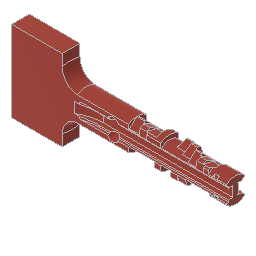
disklock family (Autodesk Fusion 360 design; units mm, degrees)
Autodesk Fusion 360 part; units mm, degrees
sketch "full profile" plane through (0, 0, 0) normal (0, 1, 0) x (1, 0, 0)
  circle A0 centre (0, 0) radius 2.98 construction
  line L0 (0, 0) -> (1.75, 0) construction
  line L1 (0, 0) -> (-1.75, 0) construction
  line L2 (1.75, 0) -> (1.75, -2.412)
  line L3 (1.75, 0) -> (1.75, 2.412)
  line L4 (-1.75, 0) -> (-1.75, 2.412)
  line L5 (-1.75, 0) -> (-1.75, -2.412)
  arc A1 (-1.75, -2.412) -> (1.75, -2.412) centre (0, 0) ccw
  arc A2 (1.75, 2.412) -> (-1.75, 2.412) centre (0, 0) ccw
  dimension "d1" = 5.96
  dimension "d2" = 1.75
  dimension "d3" = 1.75
  constraint coincident A0.centre L0.start
  constraint horizontal L0
  constraint parallel L0 L1
  constraint coincident A0 L2.end
  constraint perpendicular L0 L2
  constraint coincident A0 L3.end
  constraint perpendicular L0 L3
  constraint coincident A0 L4.end
  constraint perpendicular L1 L4
  constraint coincident A0 L5.end
  constraint perpendicular L1 L5
  measures "d1" diameter of A0
  measures "d2" distance of A0.centre L0.end
  measures "d3" distance of A0.centre L1.end
extrude "blade extrude" add sketch "full profile" along normal blind 32.5 makes body 1
sketch "bearing align" plane through (-1.75, 0, 0) normal (-1, 0, 0) x (0, -1, 0)
  line L0 (0, -2.412) -> (0, 2.412)
  line L1 (0, 2.412) -> (-32.5, 2.412)
  line L2 (-32.5, 2.412) -> (-32.5, -2.412)
  line L3 (-32.5, -2.412) -> (0, -2.412)
  line L4 (0, 0) -> (-22.5, 0) construction
  line L5 (-22.5, 0) -> (-22.5, 1) construction
  dimension "d6" = 22.5
  dimension "d7" = 1
  constraint coincident L4.start origin
  constraint perpendicular L0 L4
  constraint perpendicular L4 L5
  measures "d6" distance of L4.start L4.end
  measures "d7" distance of L4.end L5.end
sketch "bearings" plane through (0, 0, 0) normal (0, -1, 0) x (1, 0, 0)
  line L0 (1.75, -2.412) -> (1.75, 2.412)
  arc A0 (1.75, 2.412) -> (-1.75, 2.412) centre (0, 0) ccw
  line L1 (-1.75, 2.412) -> (-1.75, -2.412)
  arc A1 (-1.75, -2.412) -> (1.75, -2.412) centre (0, 0) ccw
  line L2 (1.75, 0) -> (-3.19, 0) construction
  line L3 (-3.19, 0) -> (-3.19, 1) construction
  line L4 (-3.19, 1) -> (-1.9994, 1)
  circle A2 centre (-1.9994, 1) radius 1.1906
  line L5 (-3.19, 0) -> (-3.19, -1) construction
  line L6 (-3.19, -1) -> (-1.9994, -1)
  circle A3 centre (-1.9994, -1) radius 1.1906
  line L7 (-1.9994, 1) -> (-0.8087, 1)
  line L8 (-1.9994, -1) -> (-0.8087, -1)
  dimension "d8" = 4.94
  dimension "d9" = 1
  dimension "d10" = 1.1906
  dimension "d11" = 2.3813
  dimension "d12" = 1
  dimension "d13" = 1.1906
  dimension "d14" = 2.3813
  constraint midpoint L0 L2.start
  constraint perpendicular L0 L2
  constraint perpendicular L2 L3
  constraint perpendicular L3 L4
  constraint coincident L4.end A2.centre
  constraint perpendicular L2 L5
  constraint perpendicular L5 L6
  constraint coincident L6.end A3.centre
  constraint coincident A2 L7.end
  constraint perpendicular L1 L7
  constraint coincident A3 L8.end
  constraint perpendicular L1 L8
  measures "d8" distance of L2.start L2.end
  measures "d9" distance of L2.end L3.end
  measures "d10" distance of L3.end L4.end
  measures "d11" diameter of A2
  measures "d12" distance of L2.end L5.end
  measures "d13" distance of L5.end L6.end
  measures "d14" diameter of A3
revolve "bearing 1 revolve" add sketch "bearings" angle 360 about axis through (-1.9994, 0, 1) along (1, 0, 0) separate body contours L1 A2 L7 | L1 L4 A2 L7 makes body 2
revolve "bearing 2 revolve" add sketch "bearings" angle 360 about axis through (-3.19, 0, -1) along (1, 0, 0) separate body contours L1 L6 A3 L8 | L1 A3 L8 makes body 3
move_body "bearing move" bodies 2 3 to x (1, 0, 0) y (0, 1, 0) z (0, 0, 1) at (0, 22.5, 0)
mirror "bearing mirror" about plane through (0, 0, 0) normal (1, 0, 0) of bodies 2 3 makes body 4 at (2.0624, 23.5297, 0.4055) makes body 5 at (2.0624, 22.6243, 0.1824)
combine "dimple cuts" operation cut target body 1 tool bodies 2 3 4 5
sketch "keyway profile" plane through (0, 0, 0) normal (0, -1, 0) x (1, 0, 0)
  line L0 (1.75, -2.412) -> (1.75, 2.412)
  arc A0 (1.75, 2.412) -> (-1.75, 2.412) centre (0, 0) ccw
  line L1 (-1.75, 2.412) -> (-1.75, -2.412)
  arc A1 (-1.75, -2.412) -> (1.75, -2.412) centre (0, 0) ccw
  line L2 (0, 0) -> (0.5, 0) construction
  line L3 (0.5, 0) -> (0.5, 1.035)
  line L4 (0.5, 1.035) -> (1.75, 1.035)
  line L5 (0.5, 0) -> (0.5, -1.035)
  line L6 (0.5, -1.035) -> (1.75, -1.035)
  line L7 (0, 0) -> (-0.5, 0) construction
  line L8 (-0.5, 0) -> (-0.5, 1.035)
  line L9 (-0.5, 0) -> (-0.5, -1.035)
  line L10 (-0.5, -1.035) -> (-1.75, -1.035)
  line L11 (-0.5, 1.035) -> (-1.75, 1.035)
  dimension "d22" = 0.5
  dimension "d23" = 1.035
  dimension "d24" = 1.035
  dimension "d25" = 0.5
  dimension "d26" = 1.035
  dimension "d27" = 1.035
  constraint coincident A0.centre A1.centre
  constraint perpendicular L1 L2
  constraint perpendicular L2 L3
  constraint coincident L0 L4.end
  constraint perpendicular L0 L4
  constraint perpendicular L2 L5
  constraint coincident L0 L6.end
  constraint perpendicular L0 L6
  constraint parallel L2 L7
  constraint perpendicular L7 L8
  constraint perpendicular L7 L9
  constraint coincident L1 L10.end
  constraint perpendicular L1 L10
  constraint coincident L1 L11.end
  constraint perpendicular L1 L11
  measures "d22" distance of A0.centre L2.end
  measures "d23" distance of L2.end L3.end
  measures "d24" distance of L2.end L5.end
  measures "d25" distance of A0.centre L7.end
  measures "d26" distance of L7.end L8.end
  measures "d27" distance of L7.end L9.end
extrude "keyway profile cut" cut sketch "keyway profile" against normal blind 30 contours L0 L3 L4 L5 L6 | L1 L8 L9 L10 L11 bodies 1
fillet "Fillet2" radius 8.5 2 edges at (-0.5, 30, 0) (0.5, 30, 0) on bodies 1
sketch "novel spinner warding" plane through (0, 0, 0) normal (0, 1, 0) x (1, 0, 0)
  line L0 (0, 0) -> (1.75, 0) construction
  line L1 (1.75, 0) -> (1.75, 0.99) construction
  line L2 (1.75, 0.99) -> (1.3741, 0.99)
  line L3 (1.3741, 0.99) -> (1.3741, 1.3518)
  line L4 (1.75, 0.99) -> (1.75, 1.4886)
  line L5 (1.75, 1.4886) -> (1.3741, 1.3518)
  line L6 (0, 0) -> (-1.75, 0) construction
  line L7 (-1.75, 0) -> (-1.75, -0.99) construction
  line L8 (-1.75, -0.99) -> (-1.3741, -0.99)
  line L9 (-1.3741, -0.99) -> (-1.3741, -1.3518)
  line L10 (-1.75, -0.99) -> (-1.75, -1.4886)
  line L11 (-1.75, -1.4886) -> (-1.3741, -1.3518)
  line L12 (0, 0) -> (0, 1.75) construction
  line L13 (1.3741, -0.99) -> (1.3741, -1.3518)
  line L14 (1.75, -0.99) -> (1.3741, -0.99)
  line L15 (1.75, -0.99) -> (1.75, -1.4886)
  line L16 (1.75, -1.4886) -> (1.3741, -1.3518)
  line L17 (-1.75, 1.4886) -> (-1.3741, 1.3518)
  line L18 (-1.75, 0.99) -> (-1.75, 1.4886)
  line L19 (-1.3741, 0.99) -> (-1.3741, 1.3518)
  line L20 (-1.75, 0.99) -> (-1.3741, 0.99)
  dimension "d30" = 1.75
  dimension "d31" = 0.99
  dimension "d32" = 0.3759
  dimension "d33" = 0.3618
  dimension "d34" = 0.4986
  dimension "d35" = 1.75
  dimension "d36" = 0.99
  dimension "d37" = 0.3759
  dimension "d38" = 0.3618
  dimension "d39" = 0.4986
  dimension "d40" = 1.75
  constraint coincident L0.start L6.start
  constraint horizontal L0
  constraint perpendicular L0 L1
  constraint perpendicular L1 L2
  constraint perpendicular L2 L3
  constraint perpendicular L2 L4
  constraint parallel L0 L6
  constraint perpendicular L6 L7
  constraint perpendicular L7 L8
  constraint perpendicular L8 L9
  constraint perpendicular L8 L10
  constraint perpendicular L6 L12
  constraint symmetric L1.end L12 L18.start
  constraint symmetric L2.end L12 L19.start
  constraint symmetric L3.end L12 L17.end
  constraint symmetric L4.end L12 L17.start
  constraint symmetric L7.end L12 L14.start
  constraint symmetric L8.end L12 L13.start
  constraint symmetric L9.end L12 L13.end
  constraint symmetric L10.end L12 L15.end
  measures "d30" distance of L0.start L0.end
  measures "d31" distance of L0.end L1.end
  measures "d32" distance of L1.end L2.end
  measures "d33" distance of L2.end L3.end
  measures "d34" distance of L1.end L4.end
  measures "d35" distance of L0.start L6.end
  measures "d36" distance of L6.end L7.end
  measures "d37" distance of L7.end L8.end
  measures "d38" distance of L8.end L9.end
  measures "d39" distance of L7.end L10.end
  measures "d40" distance of L0.start L12.end
extrude "spinner warding cut" cut sketch "novel spinner warding" along normal blind 29 bodies 1
fillet "Fillet1" radius 15.9 4 edges at (1.3741, 29, -1.1934) (1.3741, 29, 1.1934) (-1.3741, 29, 1.1934) (-1.3741, 29, -1.1934) on bodies 1
sketch "driver plate cut" plane through (0, 0, 0) normal (0, 1, 0) x (1, 0, 0)
  circle A0 centre (0, 0) radius 3.15 construction
  line L0 (0, 0) -> (1.82, 0) construction
  line L1 (0, 0) -> (1.758, -0.4711) construction
  line L2 (0, 0) -> (1.82, 0) construction
  line L3 (1.758, -0.4711) -> (1.0926, -2.9545)
  line L4 (0, 0) -> (-1.82, 0) construction
  line L5 (0, 0) -> (-1.758, 0.4711) construction
  line L6 (0, 0) -> (1.758, 0.4711) construction
  line L7 (0, 0) -> (1.82, 0) construction
  line L8 (0, 0) -> (-1.758, -0.4711) construction
  line L9 (1.758, 0.4711) -> (1.0926, 2.9545)
  line L10 (-1.758, -0.4711) -> (-1.0926, -2.9545)
  line L11 (-1.758, 0.4711) -> (-1.0926, 2.9545)
  line L12 (-1.758, -0.4711) -> (-1.758, 0.4711)
  line L13 (1.758, -0.4711) -> (1.758, 0.4711)
  arc A1 (-1.0926, -2.9545) -> (1.0926, -2.9545) centre (0, 0) ccw
  arc A2 (1.0926, 2.9545) -> (-1.0926, 2.9545) centre (0, 0) ccw
  circle A3 centre (0, 0) radius 3.465
  dimension "d43" = 6.3
  dimension "d44" = 1.82
  dimension "d45" = 15
  dimension "d46" = 1.82
  dimension "d47" = 1.82
  dimension "d48" = 1.82
  dimension "d49" = 15
  dimension "d50" = 1.82
  dimension "d51" = 1.82
  dimension "d52" = 6.93
  constraint coincident A0.centre L0.start
  constraint horizontal L0
  constraint horizontal L2
  constraint coincident A0 L3.end
  constraint perpendicular L1 L3
  constraint parallel L2 L4
  constraint parallel L1 L5
  constraint horizontal L7
  constraint parallel L6 L8
  constraint coincident A0 L9.end
  constraint perpendicular L6 L9
  constraint coincident A0 L10.end
  constraint perpendicular L8 L10
  constraint coincident A0 L11.end
  constraint perpendicular L5 L11
  constraint concentric A0 A3
  measures "d43" diameter of A0
  measures "d44" distance of A0.centre L0.end
  measures "d45" angle of L1 L2
  measures "d46" distance of A0.centre L1.end
  measures "d47" distance of A0.centre L4.end
  measures "d48" distance of A0.centre L5.end
  measures "d49" angle of L6 L7
  measures "d50" distance of A0.centre L6.end
  measures "d51" distance of A0.centre L8.end
  measures "d52" diameter of A3
extrude "driver plate extrude" cut sketch "driver plate cut" along normal blind 0.8 from surface at 1.9 bodies 1
sketch "tip warding clearance" plane through (0, 0, 0) normal (0, 1, 0) x (1, 0, 0)
  circle A0 centre (0, 0) radius 2.475
  circle A1 centre (0, 0) radius 3.0938
  dimension "d55" = 4.95
  dimension "d56" = 6.1875
  constraint coincident A0.centre A1.centre
  constraint concentric A0 A1
  measures "d55" diameter of A0
  measures "d56" diameter of A1
extrude "tip warding cut" cut sketch "tip warding clearance" along normal blind 3.65 bodies 1
sketch "cut 1" plane through (0, 0, 0) normal (0, 1, 0) x (1, 0, 0)
  circle A0 centre (0, 0) radius 2.98 construction
  circle A1 centre (0, 0) radius 2.1875 construction
  line L0 (0, 0) -> (1.75, 0) construction
  line L1 (1.75, 0) -> (1.75, -1.7958) construction
  line L2 (1.75, -1.7958) -> (-1.3885, -2.6367) construction
  line L3 (1.75, -1.7958) -> (-1.2492, -1.7958) construction
  line L4 (0, 0) -> (-1.75, 0) construction
  line L5 (-1.75, 0) -> (-1.75, 1.7958) construction
  line L6 (-1.75, 1.7958) -> (1.3885, 2.6367) construction
  line L7 (-1.75, 1.7958) -> (1.2492, 1.7958) construction
  line L8 (1.75, -1.3125) -> (1.75, 2.412)
  line L9 (-1.75, 1.3125) -> (-1.75, -2.412)
  line L10 (0.5662, -2.113) -> (-1.3885, -2.6367)
  line L11 (-0.5662, 2.113) -> (1.3885, 2.6367)
  arc A2 (0.5662, -2.113) -> (1.75, -1.3125) centre (0, 0) ccw
  arc A3 (-0.5662, 2.113) -> (-1.75, 1.3125) centre (0, 0) ccw
  arc A4 (1.75, 2.412) -> (1.3885, 2.6367) centre (0, 0) ccw
  arc A5 (-1.75, -2.412) -> (-1.3885, -2.6367) centre (0, 0) ccw
  circle A6 centre (0, 0) radius 3.5
  dimension "d59" = 5.96
  dimension "d60" = 4.375
  dimension "d61" = 1.75
  dimension "d62" = 15
  dimension "d63" = 1.75
  dimension "d64" = 15
  dimension "d65" = 2.98
  dimension "d66" = 2.1875
  dimension "d67" = 7
  constraint coincident A0.centre A1.centre
  constraint horizontal L0
  constraint perpendicular L0 L1
  constraint horizontal L3
  constraint coincident A0 L2.end
  constraint tangent A1 L2
  constraint coincident A1 L3.end
  constraint parallel L0 L4
  constraint perpendicular L4 L5
  constraint horizontal L7
  constraint coincident A0 L6.end
  constraint tangent A1 L6
  constraint coincident A1 L7.end
  constraint coincident A1 L8.start
  constraint coincident L1 L8.start
  constraint coincident A0 L8.end
  constraint parallel L1 L8
  constraint coincident L5 L9.start
  constraint coincident A1 L9.start
  constraint coincident A0 L9.end
  constraint parallel L5 L9
  constraint coincident A1 L10.start
  constraint coincident L2 L10.start
  constraint coincident L6 L11.start
  constraint coincident A1 L11.start
  constraint concentric A3 A6
  measures "d59" diameter of A0
  measures "d60" diameter of A1
  measures "d61" distance of A0.centre L0.end
  measures "d62" angle of L2 L3
  measures "d63" distance of A0.centre L4.end
  measures "d64" angle of L6 L7
  measures "d65" radius of A5
  measures "d66" radius of A3
  measures "d67" diameter of A6
sketch "cut 2" plane through (0, 0, 0) normal (0, 1, 0) x (1, 0, 0)
  circle A0 centre (0, 0) radius 2.98 construction
  circle A1 centre (0, 0) radius 2.1875 construction
  line L0 (0, 0) -> (1.75, 0) construction
  line L1 (0, 0) -> (-1.75, 0) construction
  line L2 (1.75, 0) -> (1.75, -1.5155) construction
  line L3 (1.75, -1.5155) -> (-0.6588, -2.9063) construction
  line L4 (1.75, -1.5155) -> (-1.5774, -1.5155) construction
  line L5 (-1.75, 0) -> (-1.75, 1.5155) construction
  line L6 (-1.75, 1.5155) -> (0.6588, 2.9063) construction
  line L7 (-1.75, 1.5155) -> (1.5774, 1.5155) construction
  line L8 (1.75, -1.3125) -> (1.75, 1.3125)
  line L9 (-1.75, 1.3125) -> (-1.75, -1.3125)
  line L10 (1.75, 1.3125) -> (1.3963, 2.6326)
  line L11 (1.75, 1.3125) -> (-1.75, 1.3125) construction
  line L12 (-1.75, -1.3125) -> (-1.3963, -2.6326)
  line L13 (-1.75, -1.3125) -> (1.75, -1.3125) construction
  line L14 (1.0937, -1.8944) -> (-0.6588, -2.9063)
  line L15 (-1.0937, 1.8944) -> (0.6588, 2.9063)
  arc A2 (1.0937, -1.8944) -> (1.75, -1.3125) centre (0, 0) ccw
  arc A3 (-1.0937, 1.8944) -> (-1.75, 1.3125) centre (0, 0) ccw
  arc A4 (1.3963, 2.6326) -> (0.6588, 2.9063) centre (0, 0) ccw
  arc A5 (-1.3963, -2.6326) -> (-0.6588, -2.9063) centre (0, 0) ccw
  circle A6 centre (0, 0) radius 3.5
  dimension "d68" = 5.96
  dimension "d69" = 4.375
  dimension "d70" = 1.75
  dimension "d71" = 1.75
  dimension "d72" = 30
  dimension "d73" = 30
  dimension "d74" = 75
  dimension "d75" = 75
  dimension "d76" = 2.98
  dimension "d77" = 2.1875
  dimension "d78" = 2.1875
  dimension "d79" = 2.98
  dimension "d80" = 7
  constraint coincident A0.centre A1.centre
  constraint horizontal L0
  constraint parallel L0 L1
  constraint perpendicular L0 L2
  constraint horizontal L4
  constraint coincident A0 L3.end
  constraint tangent A1 L3
  constraint coincident A1 L4.end
  constraint perpendicular L1 L5
  constraint horizontal L7
  constraint coincident A0 L6.end
  constraint tangent A1 L6
  constraint coincident A1 L7.end
  constraint coincident A1 L8.start
  constraint coincident L2 L8.start
  constraint coincident A1 L8.end
  constraint parallel L2 L8
  constraint coincident L5 L9.start
  constraint coincident A1 L9.start
  constraint coincident A1 L9.end
  constraint perpendicular L1 L9
  constraint horizontal L11
  constraint coincident A0 L10.end
  constraint horizontal L13
  constraint coincident A0 L12.end
  constraint coincident A1 L14.start
  constraint coincident L3 L14.start
  constraint coincident A1 L15.start
  constraint tangent A1 L15
  constraint concentric A2 A6
  measures "d68" diameter of A0
  measures "d69" diameter of A1
  measures "d70" distance of A0.centre L0.end
  measures "d71" distance of A0.centre L1.end
  measures "d72" angle of L3 L4
  measures "d73" angle of L6 L7
  measures "d74" angle of L10 L11
  measures "d75" angle of L12 L13
  measures "d76" radius of A5
  measures "d77" radius of A2
  measures "d78" radius of A3
  measures "d79" radius of A4
  measures "d80" diameter of A6
sketch "cut 3" plane through (0, 0, 0) normal (0, 1, 0) x (1, 0, 0)
  circle A0 centre (0, 0) radius 2.98 construction
  circle A1 centre (0, 0) radius 2.1875 construction
  line L0 (0, 0) -> (1.75, 0) construction
  line L1 (0, 0) -> (-1.75, 0) construction
  line L2 (1.75, 0) -> (1.75, -1.3436) construction
  line L3 (1.75, -1.3436) -> (0.1158, -2.9777) construction
  line L4 (1.75, -1.3436) -> (-1.7262, -1.3436) construction
  line L5 (-1.75, 0) -> (-1.75, -1.3436) construction
  line L6 (-1.75, -1.3436) -> (-0.1158, -2.9777) construction
  line L7 (-1.75, -1.3436) -> (1.75, -1.3436) construction
  line L8 (1.75, 0) -> (1.75, 1.3436) construction
  line L9 (1.75, 1.3436) -> (0.1158, 2.9777) construction
  line L10 (1.75, 1.3436) -> (-1.7262, 1.3436) construction
  line L11 (-1.75, 0) -> (-1.75, 1.3436) construction
  line L12 (-1.75, 1.3436) -> (-0.1158, 2.9777) construction
  line L13 (-1.75, 1.3436) -> (1.75, 1.3436) construction
  line L14 (1.75, -1.3125) -> (1.75, 1.3125)
  line L15 (-1.75, -1.3125) -> (-1.75, 1.3125)
  line L16 (-1.5468, 1.5468) -> (-0.1158, 2.9777)
  line L17 (1.5468, 1.5468) -> (0.1158, 2.9777)
  line L18 (-1.5468, -1.5468) -> (-0.1158, -2.9777)
  line L19 (1.5468, -1.5468) -> (0.1158, -2.9777)
  arc A2 (1.5468, -1.5468) -> (1.75, -1.3125) centre (0, 0) ccw
  arc A3 (-1.75, -1.3125) -> (-1.5468, -1.5468) centre (0, 0) ccw
  arc A4 (-1.5468, 1.5468) -> (-1.75, 1.3125) centre (0, 0) ccw
  arc A5 (1.75, 1.3125) -> (1.5468, 1.5468) centre (0, 0) ccw
  arc A6 (0.1158, 2.9777) -> (-0.1158, 2.9777) centre (0, 0) ccw
  arc A7 (-0.1158, -2.9777) -> (0.1158, -2.9777) centre (0, 0) ccw
  circle A8 centre (0, 0) radius 3.5
  dimension "d81" = 5.96
  dimension "d82" = 4.375
  dimension "d83" = 1.75
  dimension "d84" = 1.75
  dimension "d85" = 45
  dimension "d86" = 45
  dimension "d87" = 45
  dimension "d88" = 45
  dimension "d89" = 2.1875
  dimension "d90" = 2.1875
  dimension "d91" = 7
  constraint coincident A0.centre A1.centre
  constraint concentric A0 A1
  constraint horizontal L0
  constraint parallel L0 L1
  constraint perpendicular L0 L2
  constraint horizontal L4
  constraint coincident A0 L3.end
  constraint tangent A1 L3
  constraint coincident A1 L4.end
  constraint perpendicular L1 L5
  constraint horizontal L7
  constraint coincident A0 L6.end
  constraint tangent A1 L6
  constraint perpendicular L0 L8
  constraint horizontal L10
  constraint coincident A0 L9.end
  constraint tangent A1 L9
  constraint coincident A1 L10.end
  constraint perpendicular L1 L11
  constraint horizontal L13
  constraint coincident A0 L12.end
  constraint tangent A1 L12
  constraint coincident A1 L14.start
  constraint coincident L2 L14.start
  constraint coincident A1 L14.end
  constraint coincident L8 L14.end
  constraint coincident L5 L15.start
  constraint coincident A1 L15.start
  constraint coincident A1 L15.end
  constraint coincident L11 L15.end
  constraint coincident L12 L16.start
  constraint coincident A1 L16.start
  constraint coincident A1 L17.start
  constraint tangent A1 L17
  constraint coincident A1 L18.start
  constraint tangent A1 L18
  constraint coincident L3 L19.start
  constraint coincident A1 L19.start
  constraint concentric A6 A8
  measures "d81" diameter of A0
  measures "d82" diameter of A1
  measures "d83" distance of A0.centre L0.end
  measures "d84" distance of A0.centre L1.end
  measures "d85" angle of L3 L4
  measures "d86" angle of L6 L7
  measures "d87" angle of L9 L10
  measures "d88" angle of L12 L13
  measures "d89" radius of A3
  measures "d90" radius of A4
  measures "d91" diameter of A8
sketch "cut 4" plane through (0, 0, 0) normal (0, 1, 0) x (1, 0, 0)
  circle A0 centre (0, 0) radius 2.98 construction
  circle A1 centre (0, 0) radius 2.1875 construction
  line L0 (0, 0) -> (1.75, 0) construction
  line L1 (0, 0) -> (-1.75, 0) construction
  line L2 (-1.75, 0) -> (-1.75, -1.5155) construction
  line L3 (-1.75, -1.5155) -> (0.6588, -2.9063) construction
  line L4 (-1.75, -1.5155) -> (1.5774, -1.5155) construction
  line L5 (1.75, 0) -> (1.75, 1.5155) construction
  line L6 (1.75, 1.5155) -> (-0.6588, 2.9063) construction
  line L7 (1.75, 1.5155) -> (-1.5774, 1.5155) construction
  line L8 (-1.75, -1.3125) -> (-1.75, 1.3125)
  line L9 (1.75, 1.3125) -> (1.75, -1.3125)
  line L10 (1.75, -1.3125) -> (1.3963, -2.6326)
  line L11 (1.75, -1.3125) -> (-1.75, -1.3125) construction
  line L12 (-1.75, 1.3125) -> (-1.3963, 2.6326)
  line L13 (-1.75, 1.3125) -> (1.75, 1.3125) construction
  line L14 (-1.0938, -1.8944) -> (0.6588, -2.9063)
  line L15 (1.0937, 1.8944) -> (-0.6588, 2.9063)
  arc A2 (1.75, 1.3125) -> (1.0938, 1.8944) centre (0, 0) ccw
  arc A3 (-1.75, -1.3125) -> (-1.0938, -1.8944) centre (0, 0) ccw
  arc A4 (0.6588, -2.9063) -> (1.3963, -2.6326) centre (0, 0) ccw
  arc A5 (-0.6588, 2.9063) -> (-1.3963, 2.6326) centre (0, 0) ccw
  circle A6 centre (0, 0) radius 3.5
  dimension "d92" = 5.96
  dimension "d93" = 4.375
  dimension "d94" = 1.75
  dimension "d95" = 1.75
  dimension "d96" = 30
  dimension "d97" = 30
  dimension "d98" = 75
  dimension "d99" = 75
  dimension "d100" = 2.1875
  dimension "d101" = 2.98
  dimension "d102" = 7
  constraint coincident A0.centre A1.centre
  constraint horizontal L0
  constraint parallel L0 L1
  constraint perpendicular L1 L2
  constraint horizontal L4
  constraint coincident A0 L3.end
  constraint tangent A1 L3
  constraint coincident A1 L4.end
  constraint perpendicular L0 L5
  constraint horizontal L7
  constraint coincident A0 L6.end
  constraint tangent A1 L6
  constraint coincident A1 L7.end
  constraint coincident A1 L8.start
  constraint coincident L2 L8.start
  constraint coincident A1 L8.end
  constraint perpendicular L1 L8
  constraint coincident A1 L9.start
  constraint coincident L5 L9.start
  constraint coincident A1 L9.end
  constraint perpendicular L7 L9
  constraint horizontal L11
  constraint coincident A0 L10.end
  constraint horizontal L13
  constraint coincident A0 L12.end
  constraint coincident A1 L14.start
  constraint tangent A1 L14
  constraint coincident A1 L15.start
  constraint tangent A1 L15
  constraint concentric A1 A6
  measures "d92" diameter of A0
  measures "d93" diameter of A1
  measures "d94" distance of A0.centre L0.end
  measures "d95" distance of A0.centre L1.end
  measures "d96" angle of L3 L4
  measures "d97" angle of L6 L7
  measures "d98" angle of L10 L11
  measures "d99" angle of L12 L13
  measures "d100" radius of A3
  measures "d101" radius of A4
  measures "d102" diameter of A6
sketch "cut 5" plane through (0, 0, 0) normal (0, 1, 0) x (1, 0, 0)
  circle A0 centre (0, 0) radius 2.98 construction
  circle A1 centre (0, 0) radius 2.1875 construction
  line L0 (0, 0) -> (1.75, 0) construction
  line L1 (0, 0) -> (-1.75, 0) construction
  line L2 (-1.75, 0) -> (-1.75, -1.7958) construction
  line L3 (-1.75, -1.7958) -> (1.3885, -2.6367) construction
  line L4 (-1.75, -1.7958) -> (1.2492, -1.7958) construction
  line L5 (1.75, 0) -> (1.75, 1.7958) construction
  line L6 (1.75, 1.7958) -> (-1.3885, 2.6367) construction
  line L7 (1.75, 1.7958) -> (-1.2492, 1.7958) construction
  line L8 (-1.75, -1.3125) -> (-1.75, 2.412)
  line L9 (1.75, 1.3125) -> (1.75, -2.412)
  line L10 (-0.5662, -2.113) -> (1.3885, -2.6367)
  line L11 (0.5662, 2.113) -> (-1.3885, 2.6367)
  arc A2 (-1.75, -1.3125) -> (-0.5662, -2.113) centre (0, 0) ccw
  arc A3 (1.75, 1.3125) -> (0.5662, 2.113) centre (0, 0) ccw
  arc A4 (-1.3885, 2.6367) -> (-1.75, 2.412) centre (0, 0) ccw
  arc A5 (1.3885, -2.6367) -> (1.75, -2.412) centre (0, 0) ccw
  circle A6 centre (0, 0) radius 3.5
  dimension "d103" = 5.96
  dimension "d104" = 4.375
  dimension "d105" = 1.75
  dimension "d106" = 1.75
  dimension "d107" = 15
  dimension "d108" = 15
  dimension "d109" = 2.98
  dimension "d110" = 2.1875
  dimension "d111" = 7
  constraint coincident A0.centre A1.centre
  constraint horizontal L0
  constraint parallel L0 L1
  constraint perpendicular L1 L2
  constraint horizontal L4
  constraint coincident A0 L3.end
  constraint tangent A1 L3
  constraint coincident A1 L4.end
  constraint perpendicular L0 L5
  constraint horizontal L7
  constraint coincident A0 L6.end
  constraint tangent A1 L6
  constraint coincident A1 L7.end
  constraint coincident A1 L8.start
  constraint coincident L2 L8.start
  constraint coincident A0 L8.end
  constraint parallel L2 L8
  constraint coincident A1 L9.start
  constraint coincident L5 L9.start
  constraint coincident A0 L9.end
  constraint parallel L5 L9
  constraint coincident L3 L10.start
  constraint coincident A1 L10.start
  constraint coincident A1 L11.start
  constraint tangent A1 L11
  constraint concentric A5 A6
  measures "d103" diameter of A0
  measures "d104" diameter of A1
  measures "d105" distance of A0.centre L0.end
  measures "d106" distance of A0.centre L1.end
  measures "d107" angle of L3 L4
  measures "d108" angle of L6 L7
  measures "d109" radius of A5
  measures "d110" radius of A3
  measures "d111" diameter of A6
sketch "cut 6" plane through (0, 0, 0) normal (0, 1, 0) x (1, 0, 0)
  circle A0 centre (0, 0) radius 2.1875
  circle A1 centre (0, 0) radius 3.5
  dimension "d112" = 4.375
  dimension "d113" = 7
  constraint coincident A0.centre A1.centre
  constraint concentric A0 A1
  measures "d112" diameter of A0
  measures "d113" diameter of A1
extrude "1" cut sketch "cut 1" along normal blind 1 and the other way blind 0.65 from surface at 4 bodies 1
extrude "2" cut sketch "cut 2" along normal mid plane 2 from surface at 5.6 bodies 1
extrude "3" cut sketch "cut 3" along normal mid plane 2 from surface at 7.2 bodies 1
extrude "4" cut sketch "cut 4" along normal mid plane 2 from surface at 8.8 bodies 1
extrude "5" cut sketch "cut 5" along normal mid plane 2 from surface at 10.4 bodies 1
extrude "6" cut sketch "cut 6" along normal mid plane 2 from surface at 12 bodies 1
extrude "7" [suppressed]
extrude "8" cut sketch "cut 1" along normal mid plane 2 from surface at 15.2 bodies 1
extrude "9" cut sketch "cut 2" along normal mid plane 2 from surface at 16.8 bodies 1
extrude "10" cut sketch "cut 3" along normal mid plane 2 from surface at 18.4 bodies 1
sketch "bow" plane through (0, 32.5, 0) normal (0, 1, 0) x (-1, 0, 0)
  line L0 (-1.75, 2.412) -> (-1.75, -2.412)
  arc A0 (-1.75, -2.412) -> (1.75, -2.412) centre (0, 0) ccw
  line L1 (1.75, -2.412) -> (1.75, 2.412)
  arc A1 (1.75, 2.412) -> (-1.75, 2.412) centre (0, 0) ccw
  line L2 (0, 0) -> (0, 2.98) construction
  line L3 (0, 0) -> (0, -2.98) construction
  line L4 (0, 2.98) -> (1.75, 2.98) construction
  line L5 (1.75, 2.98) -> (1.75, 8)
  line L6 (1.75, 8) -> (-1.75, 8)
  line L7 (0, -2.98) -> (-1.75, -2.98) construction
  line L8 (-1.75, -2.98) -> (-1.75, -8) construction
  line L9 (-1.75, 8) -> (-1.75, -8)
  line L10 (-1.75, -8) -> (1.75, -8)
  line L11 (1.75, -8) -> (1.75, 2.98)
  dimension "d147" = 1.75
  dimension "d148" = 5.02
  dimension "d149" = 3.5
  dimension "d150" = 1.75
  dimension "d151" = 5.02
  constraint coincident A0.centre A1.centre
  constraint midpoint A1 L2.end
  constraint midpoint A0 L3.end
  constraint perpendicular L2 L4
  constraint perpendicular L4 L5
  constraint perpendicular L5 L6
  constraint perpendicular L3 L7
  constraint perpendicular L7 L8
  constraint perpendicular L5 L10
  constraint perpendicular L4 L11
  measures "d147" distance of L2.end L4.end
  measures "d148" distance of L4.end L5.end
  measures "d149" distance of L5.end L6.end
  measures "d150" distance of L3.end L7.end
  measures "d151" distance of L7.end L8.end
extrude "bow extrude" add sketch "bow" along normal blind 10 bodies 1
fillet "Fillet3" radius 3 2 edges at (0, 32.5, 2.98) (0, 32.5, -2.98) on bodies 1
equation "d2 = ( 3.5 * 0.5 ) * 1 mm"
equation "d3 = d2"
equation "d9 = d7"
equation "d10 = 0.5 * ( ( 3 / 32 ) * 1 in )"
equation "d11 = ( 3 / 32 ) * 1 in"
equation "d12 = d9"
equation "d13 = d10"
equation "d14 = d11"
equation "d18 = d6"
equation "d23 = ( 1.9 / 2 ) * 1 mm + 0.085 mm"
equation "d24 = d23"
equation "d25 = d22"
equation "d26 = d23"
equation "d27 = d23"
equation "d30 = d2"
equation "d32 = ( 0.4 * cos(20 deg) ) * 1 mm"
equation "d33 = ( 0.4 * sin(20 deg) ) * 1 mm + 0.225 mm"
equation "d34 = ( ( 0.4 * sin(20 deg) ) * 1 mm + 0.225 mm ) + ( ( 0.4 * sin(20 deg) ) * 1 mm )"
equation "d35 = d30"
equation "d36 = d31"
equation "d37 = d32"
equation "d38 = d33"
equation "d39 = d34"
equation "d40 = d2"
equation "d44 = ( 3.64 * 0.5 ) * 1 mm"
equation "d46 = d44"
equation "d47 = d44"
equation "d48 = d44"
equation "d49 = d45"
equation "d50 = d44"
equation "d51 = d44"
equation "d52 = d43 * 1.1"
equation "d56 = d55 * 1.25"
equation "d57 = offset + cut_spacing - cut_width + d219"
equation "d59 = d1"
equation "d61 = d2"
equation "d63 = d2"
equation "d64 = d62"
equation "d68 = d1"
equation "d69 = d60"
equation "d70 = d2"
equation "d71 = d2"
equation "d73 = d72"
equation "d75 = d74"
equation "d80 = d67"
equation "d81 = d1"
equation "d82 = d60"
equation "d83 = d2"
equation "d84 = d2"
equation "d86 = d85"
equation "d87 = d85"
equation "d88 = d85"
equation "d91 = d67"
equation "d92 = d1"
equation "d93 = d60"
equation "d94 = d2"
equation "d95 = d2"
equation "d96 = d72"
equation "d97 = d72"
equation "d98 = d74"
equation "d99 = d74"
equation "d102 = d67"
equation "d103 = d1"
equation "d104 = d60"
equation "d105 = d2"
equation "d106 = d2"
equation "d107 = d62"
equation "d108 = d62"
equation "d111 = d67"
equation "d112 = d60"
equation "d113 = d67"
equation "d114 = offset + ( cut_spacing * 1 )"
equation "d115 = cut_width"
equation "d119 = offset + ( cut_spacing * 2 )"
equation "d120 = cut_width"
equation "d122 = offset + ( cut_spacing * 3 )"
equation "d123 = cut_width"
equation "d125 = offset + ( cut_spacing * 4 )"
equation "d126 = cut_width"
equation "d128 = offset + ( cut_spacing * 5 )"
equation "d129 = cut_width"
equation "d131 = offset + ( cut_spacing * 6 )"
equation "d132 = cut_width"
equation "d134 = offset + ( cut_spacing * 8 )"
equation "d135 = cut_width"
equation "d137 = offset + ( cut_spacing * 9 )"
equation "d138 = cut_width"
equation "d140 = offset + ( cut_spacing * 10 )"
equation "d141 = cut_width"
equation "d147 = d2"
equation "d148 = 8 mm - ( 0.5 * 5.96 ) * 1 mm"
equation "d149 = d2 * 2"
equation "d150 = d2"
equation "d151 = d148"
equation "d156 = 2.2 mm + ( 1.5 * 7 mm )"
equation "cut_spacing = 1.6 mm"
equation "offset = 2.4 mm"
equation "cut_width = 1 mm" comment "value is double"
equation "d219 = cut_width - 0.35 mm"
named bodies: "blade", "bearing 1", "bearing 2", "bearing 3", "bearing 4"
